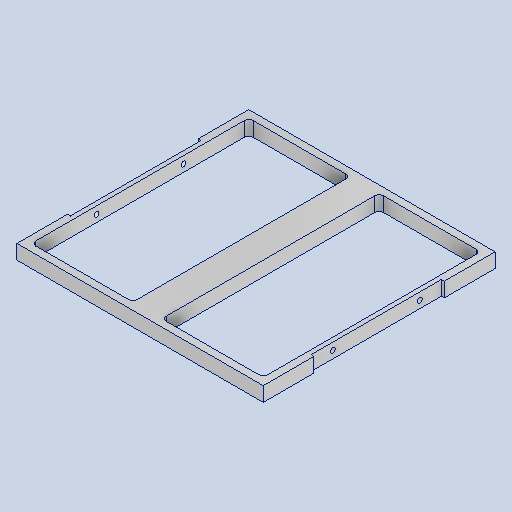
# Autodesk Inventor part: Mirror_shell3
Saved by Autodesk Inventor 2023 (Build 270158000, 158)
## iProperties
Created: 2023-04-13
Part Number: Mirror_shell3
Material: Aluminum 6061
Document SubType Name: Modeling
Designer: ASARe-DAQ-PC
Density: 2.7 g/cm^3
Appearance: Aluminum - Flat
Mass: 157.785 g
Surface Area: 271.429 cm^2
Volume: 58.4391 cm^3
Author: ASARe-DAQ-PC
Autodesk Inventor part; units mm, degrees
ref_plane "YZ Plane" through (0, 0, 0) normal (1, 0, 0) x (0, 1, 0)
ref_plane "XZ Plane" through (0, 0, 0) normal (0, 1, 0) x (-1, 0, 0)
sketch "Sketch1" plane through (0, 0, 0) normal (0, 1, 0) x (-1, 0, 0)
  line L0 (0, 0) -> (170, 0)
  line L1 (170, 0) -> (170, -160)
  line L2 (170, -160) -> (0, -160)
  line L3 (0, -160) -> (0, 0)
  line L4 (5, -5) -> (165, -5)
  line L5 (165, -5) -> (165, -155)
  line L6 (165, -155) -> (5, -155)
  line L7 (5, -155) -> (5, -5)
  line L8 (95, -5) -> (75, -5)
  line L9 (75, -5) -> (75, -155)
  line L10 (75, -155) -> (95, -155)
  line L11 (95, -155) -> (95, -5)
  point P0 (85, -5)
  point P1 (85, 0)
  point P2 (95, -155)
  point P3 (75, -5)
  dimension "d0" = 170
  dimension "d1" = 160
  dimension "d2" = 5
  dimension "d5" = 20
  constraints: 24 end point, 6 parallel, 3 perpendicular, 2 horizontal, 2 midpoint, 2 point on line, 1 vertical alignment, 3 other
  measures "d0" distance of L0.start L0.end
  measures "d1" distance of L0.end L1.end
  measures "d2" distance between parallel lines of L3 L7
  measures "d5" distance between parallel lines of L11 L9
extrude "Extrusion1" add sketch "Sketch1" along normal blind 10 contours L0 L1 L2 L3 | L4 L11 L6 L9
fillet "Fillet1" radius 3 8 edges at (-165, 5, -5) (-95, 5, -5) (-5, 5, -5) (-5, 5, -155) (-75, 5, -155) (-95, 5, -155) (-75, 5, -5) (-165, 5, -155)
sketch "Sketch2" plane through (-5, 0, -152) normal (-1, 0, 0) x (0, 0, 1)
  line L0 (144, 10) -> (144, 0) construction
  line L1 (144, 5) -> (0, 5) construction
  line L2 (0, 0) -> (0, 10) construction
  line L3 (147, 0) -> (147, 10) construction
  line L4 (-3, 10) -> (-3, 0) construction
  point P0 (152, 0)
  point P1 (102, 5)
  point P2 (42, 5)
  point P3 (-3, 5)
  dimension "d20" = 45
  dimension "d21" = 45
  constraints: 3 midpoint, 2 end point, 2 point on line
  measures "d20" distance from line of L3 point (102, 5)
  measures "d21" distance of point (-3, 5) point (42, 5)
hole "Hole1" at (-5, 5, -50) at (-5, 5, -110) direction (1, 0, 0) diameter 3.5 end through all
sketch "Sketch5" plane through (0, 0, 0) normal (1, 0, 0) x (0, 0, -1)
  line L0 (8, 10) -> (152, 10) projected
  line L1 (8, 0) -> (152, 0) projected
  line L2 (35, 10) -> (125, 10)
  line L3 (125, 10) -> (125, 0)
  line L4 (125, 0) -> (35, 0)
  line L5 (35, 0) -> (35, 10)
  line L6 (0, 0) -> (0, 10) projected
  point P0 (0, 5)
  dimension "d37" = 90
  dimension "d38" = 35
  constraints: 8 end point, 2 parallel, 2 point on line, 1 horizontal, 1 midpoint, 1 perpendicular
  measures "d37" distance between parallel lines of L3 L5
  measures "d38" distance from line of point (0, 5) L5
extrude "Extrusion5" cut sketch "Sketch5" against normal blind 2
sketch "Sketch6" plane through (-170, 0, -160) normal (-1, 0, 0) x (0, 0, 1)
  line L0 (8, 0) -> (152, 0) projected
  line L1 (125, 10) -> (35, 10) projected
  line L2 (35, 0) -> (125, 0)
  line L3 (125, 0) -> (125, 10)
  line L4 (125, 10) -> (35, 10)
  line L5 (35, 10) -> (35, 0)
  line L6 (0, 0) -> (0, 10) projected
  point P0 (160, 0)
  dimension "d41" = 90
  dimension "d42" = 35
  constraints: 8 end point, 2 parallel, 2 point on line, 1 horizontal, 1 perpendicular
  measures "d41" distance between parallel lines of L3 L5
  measures "d42" distance between parallel lines of L6 L5
extrude "Extrusion6" cut sketch "Sketch6" against normal blind 2
ref_plane "Work Plane2" through (-85, 0, 0) normal (1, 0, 0) x (0, 0, -1)
mirror "Mirror2" about plane through (-85, 0, 0) normal (1, 0, 0) of "Hole1"
body "Solid1"
